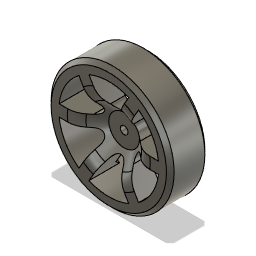
Hjul v2 (Autodesk Fusion 360 design; units mm, degrees)
Autodesk Fusion 360 part; units mm, degrees
sketch "Sketch1" plane through (0, 0, 0) normal (0, 0, 1) x (1, 0, 0)
  circle A0 centre (0, 0) radius 16
  circle A1 centre (0, 0) radius 1
  circle A2 centre (0, 0) radius 4
  circle A3 centre (0, 0) radius 13
  line L0 (0, 0) -> (16, 0) construction
  line L1 (3.708099, -1.5) -> (3.708099, 1.5) construction
  line L2 (12.913172, 1.5) -> (12.913172, -1.5) construction
  line L3 (3.708099, 1.5) -> (12.913172, 1.5)
  line L4 (3.708099, -1.5) -> (12.913172, -1.5)
  line L5 (0.555012, 3.961308) -> (5.157548, 11.933135)
  line L6 (3.153088, 2.461308) -> (7.755624, 10.433135)
  line L7 (-3.153088, 2.461308) -> (-7.755624, 10.433135)
  line L8 (-0.555012, 3.961308) -> (-5.157548, 11.933135)
  line L9 (-3.708099, -1.5) -> (-12.913172, -1.5)
  line L10 (-3.708099, 1.5) -> (-12.913172, 1.5)
  line L11 (-0.555012, -3.961308) -> (-5.157548, -11.933135)
  line L12 (-3.153088, -2.461308) -> (-7.755624, -10.433135)
  line L13 (3.153088, -2.461308) -> (7.755624, -10.433135)
  line L14 (0.555012, -3.961308) -> (5.157548, -11.933135)
  dimension "d1" = 32
  dimension "d2" = 2
  dimension "d3" = 8
  dimension "d4" = -3
  dimension "d5" = 3
  dimension "d7" = 360
  constraint coincident A0.centre A1.centre
  constraint concentric A1 A2
  constraint coincident A0 L0.end
  constraint horizontal L0
  constraint vertical L1
  constraint parallel L1 L2
  constraint equal L1 L2
  measures "d1" diameter of A0
  measures "d2" diameter of A1
  measures "d3" diameter of A2
extrude "Extrude1" add sketch "Sketch1" along normal blind 10 contours A0 picked at (-12.964551, -7.485087) makes body 1
extrude "Extrude2" add sketch "Sketch1" along normal blind 6 and the other way blind -4 separate body contours A2 picked at (2.232956, -1.995173) makes body 2
extrude "Extrude3" add sketch "Sketch1" along normal blind 10 and the other way blind -4 contours A2 A3 L3 L4 | A2 A3 L5 L6 | A2 A3 L13 L14 | A2 A3 L7 L8 | A2 A3 L11 L12 | A2 A3 L9 L10 picked at (6.976198, -0.504123) picked at (4.996781, 8.654678) picked at (4.996781, -8.654678) picked at (-4.996781, 8.654678) picked at (-4.996781, -8.654678) picked at (-9.993562, 0) bodies 1 2
draft "Draft1" angle 50 neutral plane through (0, 0, 6) pull (0, 0, 1) 6 faces at (-2.559826, 3.073644, 8.666667) (1.697159, 3.622106, 8.666667) (3.909136, 0.847737, 7.333333) (2.931598, -2.721348, 8.666667) (-0.723644, -3.933998, 8.666667) (-3.909136, -0.847737, 8.666667) on bodies 1
fillet "Fillet1" radius 5.5 6 edges at (4.383507, 7.592457, 10) (-4.383507, 7.592457, 10) (-8.767014, 0, 10) (-4.383507, -7.592457, 10) (4.383507, -7.592457, 10) (8.767014, 0, 10) on bodies 1
chamfer "Chamfer1" distance 2 angle 45 5 edges at (-6.5, -11.25833, 4) (-13, 0, 4) (-6.5, 11.25833, 4) (13, 0, 4) (6.5, -11.25833, 4) on bodies 1
fillet "Fillet2" radius 2 12 edges at (-3.708099, 1.5, 5) (-3.153088, 2.461308, 5) (-0.555012, 3.961308, 5) (0.555012, 3.961308, 5) (3.153088, 2.461308, 5) (3.708099, 1.5, 5) (3.708099, -1.5, 5) (3.153088, -2.461308, 5) (0.555012, -3.961308, 5) (-0.555012, -3.961308, 5) (-3.153088, -2.461308, 5) (-3.708099, -1.5, 5) on bodies 1
chamfer "Chamfer2" distance 1 angle 45 2 edges at (-14.917238, -5.785847, 10) (-14.917238, -5.785847, 0) on bodies 1
equation "d1 = ( 16 * 2 ) * 1 mm"
